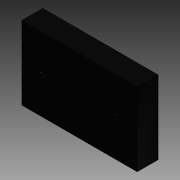
# Autodesk Inventor part: Batteriehalter_6AA
Saved by Autodesk Inventor 2015 (Build 190159000, 159)
## iProperties
Created: 2015-02-25
Part Number: Batteriehalter_6AA
Material: PBT-Kunststoff
Document SubType Name: Modeling
Designer: TowerSebi
Density: 1.31 g/cm^3
Appearance: Glatt - schwarz
GlobalPropertyList: <PropertyList/>
Author: TowerSebi
Autodesk Inventor part; units mm, degrees
ref_plane "YZ Plane" through (0, 0, 0) normal (1, 0, 0) x (0, 1, 0)
ref_plane "XZ Plane" through (0, 0, 0) normal (0, 1, 0) x (-1, 0, 0)
ref_plane "XY Plane" through (0, 0, 0) normal (0, 0, 1) x (1, 0, 0)
sketch "Skizze1" plane through (0, 0, 0) normal (0, 1, 0) x (-1, 0, 0)
  line L0 (0, 0) -> (90.25, 0)
  line L1 (90.25, 0) -> (90.25, 57.5)
  line L2 (90.25, 57.5) -> (0, 57.5)
  line L3 (0, 57.5) -> (0, 0)
  dimension "d0" = 90.25
  dimension "d1" = 57.5
  constraints: 8 end point, 2 parallel, 1 horizontal, 1 perpendicular
  measures "d0" distance of L1.end L2.end
  measures "d1" distance of L2.end L0.start
extrude "Extrusion1" add sketch "Skizze1" along normal blind 16.5
hole "Bohrung1" at (-16.5, 0, 28.75) direction (0, 1, 0) diameter 4 end through all
hole "Bohrung2" at (-73.75, 0, 28.75) direction (0, 1, 0) diameter 4 end through all
